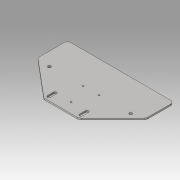
# Autodesk Inventor part: track side panel V1
Saved by Autodesk Inventor 2016 (Build 200138000, 138)
## iProperties
Created: 2015-10-10
Part Number: track side panel V1
Material: Generic
Document SubType Name: Modeling
Designer: Delta
Density: 1 g/cm^3
Appearance: Default
Author: Delta
Autodesk Inventor part; units mm, degrees
ref_plane "YZ Plane" through (0, 0, 0) normal (1, 0, 0) x (0, 1, 0)
ref_plane "XZ Plane" through (0, 0, 0) normal (0, 1, 0) x (-1, 0, 0)
ref_plane "XY Plane" through (0, 0, 0) normal (0, 0, 1) x (1, 0, 0)
sketch "Sketch1" plane through (0, 0, 0) normal (0, 1, 0) x (-1, 0, 0)
  line L0 (-77.6185, -139.5068) -> (-293.5185, -139.5068)
  line L1 (-293.5185, -139.5068) -> (-293.5185, -291.9068)
  line L2 (-293.5185, -291.9068) -> (-77.6185, -291.9068)
  line L3 (-77.6185, -291.9068) -> (-77.6185, -139.5068)
  point P0 (0, 0)
  dimension "d0" = 215.9
  dimension "d1" = 152.4
  constraints: 8 end point, 2 parallel, 1 horizontal, 1 perpendicular
  measures "d0" distance of L2.end L1.end
  measures "d1" distance of L1.end L0.end
extrude "Extrusion1" add sketch "Sketch1" along normal blind 3.175
sketch "Sketch2" plane through (0, 3.175, 0) normal (0, 1, 0) x (1, 0, 0)
  line L0 (77.6185, 291.9068) -> (77.6185, 139.5068) projected
  line L1 (77.6185, 139.5068) -> (293.5185, 139.5068) projected
  line L2 (293.5185, 139.5068) -> (293.5185, 291.9068) projected
  line L3 (293.5185, 291.9068) -> (77.6185, 291.9068) projected
  point P0 (0, 0)
  point P1 (156.9685, 165.5068)
  point P2 (104.9685, 218.5068)
  point P3 (269.9685, 218.5068)
  point P4 (221.9685, 165.5068)
  dimension "d4" = 144.35
  dimension "d5" = 26
  dimension "d7" = 79
  dimension "d19" = 27.35
  dimension "d20" = 79
  dimension "d21" = 26
  dimension "d22" = 79.35
  dimension "d23" = 192.35
  measures "d4" distance from line of L0 point (221.968, 165.507)
  measures "d5" distance from line of L1 point (221.968, 165.507)
  measures "d7" distance from line of L1 point (269.968, 218.507)
  measures "d19" distance from line of L0 point (104.968, 218.507)
  measures "d20" distance from line of L1 point (104.968, 218.507)
  measures "d21" distance from line of L1 point (156.968, 165.507)
  measures "d22" distance from line of L0 point (156.968, 165.507)
  measures "d23" distance from line of L0 point (269.968, 218.507)
hole "Hole1" at (156.9685, 3.175, -165.5068) at (104.9685, 3.175, -218.5068) at (269.9685, 3.175, -218.5068) at (221.9685, 3.175, -165.5068) direction (0, -1, 0) diameter 6 end through all
sketch "Sketch3" plane through (0, 3.175, 0) normal (0, 1, 0) x (1, 0, 0)
  line L0 (155.9994, 158.0068) -> (221.9685, 158.0068)
  circle A0 centre (221.9685, 165.5068) radius 3 projected
  circle A1 centre (104.3905, 218.5068) radius 3
  circle A2 centre (156.9685, 165.5068) radius 3 projected
  line L1 (153.2717, 158.9097) -> (79.8868, 220.4869)
  line L2 (77.6185, 139.5068) -> (293.5185, 139.5068)
  line L3 (293.5185, 229.1509) -> (293.5185, 276.0791)
  line L4 (293.5185, 291.9068) -> (77.6185, 291.9068)
  line L5 (77.6185, 291.9068) -> (77.6185, 139.5068)
  arc A3 (153.2717, 158.9097) -> (155.9994, 158.0068) centre (156.9685, 165.5068) ccw
  line L6 (96.6333, 206.4349) -> (77.6185, 222.3902)
  line L7 (48.2791, 233.5068) -> (391.5458, 233.5068) construction
  arc A4 (221.9685, 158.0068) -> (227.8466, 160.8487) centre (221.9685, 165.5068) ccw
  line L8 (227.8466, 160.8487) -> (291.6586, 224.6608)
  line L9 (293.5185, 226.5206) -> (293.5185, 282.4291)
  line L10 (293.5185, 139.5068) -> (293.5185, 291.9068) projected
  line L11 (287.1685, 282.4291) -> (83.9685, 282.4291)
  line L12 (77.6185, 276.0791) -> (77.6185, 225.3513)
  line L13 (77.6185, 291.9068) -> (77.6185, 139.5068) projected
  arc A5 (293.5185, 276.0791) -> (287.1685, 282.4291) centre (287.1685, 276.0791) ccw
  arc A6 (83.9685, 282.4291) -> (77.6185, 276.0791) centre (83.9685, 276.0791) ccw
  arc A7 (77.6185, 225.3513) -> (79.8868, 220.4869) centre (83.9685, 225.3513) ccw
  arc A8 (291.6586, 224.6608) -> (293.5185, 229.1509) centre (287.1685, 229.1509) ccw
  point P0 (0, 0)
  point P1 (77.6185, 282.4291)
  point P2 (77.6185, 160.8487)
  dimension "d24" = 7.5
  dimension "d40" = 98.7582
  dimension "d72" = 6
  dimension "d93" = 7.5
  dimension "d96" = 52.578
  dimension "d99" = 135
  dimension "d100" = 6.35
  dimension "d101" = 6.35
  dimension "d102" = 6.35
  dimension "d103" = 6.35
  dimension "d104" = 140
  constraints: 24 end point, 15 point on line, 12 point on circle, 8 tangent, 7 centre point, 4 horizontal, 2 coincident, 2 parallel, 1 collinear, 1 perpendicular
  measures "d24" distance from line of L0 A0.centre
  measures "d40" distance of L1.start L6.end
  measures "d72" diameter of A2
  measures "d93" radius of A4
  measures "d96" horizontal distance of A1.centre A3.centre
  measures "d99" angle of L0 L8
  measures "d100" radius of A5
  measures "d101" radius of A6
  measures "d102" radius of A7
  measures "d103" radius of A8
  measures "d104" angle of L0 L1
extrude "Extrusion3" cut sketch "Sketch3" against normal blind 25.4 contours L0 A4 L8 A8 L9 L10 L2 L5 L6 L1 A3 | L6 L5 A7 | A5 L11 A6 L5 L4 L10 L9
sketch "Sketch7" plane through (0, 3.175, 0) normal (0, 1, 0) x (1, 0, 0)
  circle A0 centre (156.9685, 165.5068) radius 3 projected
  line L0 (155.9994, 158.0068) -> (221.9685, 158.0068) projected
  circle A1 centre (156.9685, 178.0036) radius 2.9972
  line L1 (153.9713, 178.0036) -> (153.9713, 165.3773)
  line L2 (159.9657, 178.0043) -> (159.9685, 165.5075)
  circle A2 centre (221.9713, 178.0036) radius 2.9972
  circle A3 centre (221.9685, 165.5068) radius 3 projected
  line L3 (218.9741, 178.016) -> (218.9741, 165.3232)
  line L4 (224.9685, 178.0036) -> (224.9685, 165.5068)
  point P0 (0, 0)
  point P1 (218.9685, 165.5082)
  dimension "d76" = 5.9944
  dimension "d77" = 12.4968
  dimension "d78" = 5.9944
  dimension "d79" = 12.4968
  dimension "d88" = 6
  constraints: 9 point on circle, 8 end point, 3 vertical, 2 centre point, 1 tangent, 3 other
  measures "d76" diameter of A1
  measures "d77" distance of A0.centre A1.centre
  measures "d78" diameter of A2
  measures "d79" distance of A3.centre A2.centre
  measures "d88" diameter of A0
extrude "Extrusion4" cut sketch "Sketch7" against normal blind 25.4 contours A0 L1 A1 L2 | A1
sketch "Sketch8" plane through (0, 3.175, 0) normal (0, 1, 0) x (1, 0, 0)
  arc A0 (224.9685, 178.0036) -> (218.9741, 177.9913) centre (221.9713, 178.0036) ccw
  circle A1 centre (221.9685, 165.5068) radius 3
  line L0 (218.9741, 178.016) -> (218.9741, 165.3232)
  line L1 (224.9685, 178.0036) -> (224.9685, 165.5068)
  point P0 (0, 0)
  point P1 (218.9685, 165.5082)
  dimension "d82" = 5.9944
  dimension "d83" = 12.4968
  constraints: 6 point on circle, 4 end point, 2 centre point, 2 vertical, 1 point on line
  measures "d82" diameter of A0
  measures "d83" distance of A1.centre A0.centre
extrude "Extrusion5" cut sketch "Sketch8" against normal blind 25.4 contours L1 A1 L0 A0 | A1 L0 picked at (221.9464, 164.5591)
sketch "Sketch9" plane through (0, 3.175, 0) normal (0, 1, 0) x (1, 0, 0)
  point P0 (0, 0)
sketch "Sketch5" plane through (0, 3.175, 0) normal (0, 1, 0) x (1, 0, 0)
  circle A0 centre (104.9685, 218.5068) radius 3 projected
  circle A1 centre (104.9685, 218.5068) radius 22.225
  circle A2 centre (156.9685, 165.5068) radius 3 projected
  circle A3 centre (156.9685, 165.5068) radius 22.225
  circle A4 centre (221.9685, 165.5068) radius 3 projected
  circle A5 centre (221.9685, 165.5068) radius 22.225
  circle A6 centre (269.9685, 218.5068) radius 3 projected
  circle A7 centre (269.9685, 218.5068) radius 22.225
  line L0 (155.9994, 158.0068) -> (221.9685, 158.0068) projected
  line L1 (274.8943, 278.8204) -> (98.1742, 278.8204) projected
  arc A8 (224.9685, 178.0036) -> (218.9741, 178.016) centre (221.9713, 178.0036) ccw projected
  point P0 (0, 0)
  point P1 (205.7185, 218.5096)
  point P2 (189.4685, 178.0036)
  point P3 (173.2185, 218.5096)
  dimension "d45" = 44.45
  dimension "d47" = 44.45
  dimension "d48" = 44.45
  dimension "d49" = 44.45
  dimension "d50" = 60.5028
  dimension "d52" = 65
  dimension "d53" = 16.25
  dimension "d54" = 16.25
  dimension "d55" = 60.5028
  dimension "d58" = 52
  dimension "d62" = 32.5
  dimension "d95" = 60.3136
  dimension "d125" = 0
  constraints: 4 centre point, 4 coincident
  measures "d45" diameter of A1
  measures "d47" diameter of A3
  measures "d48" diameter of A5
  measures "d49" diameter of A7
  measures "d50" distance from line of L0 point (173.218, 218.51)
  measures "d52" distance of A5.centre A3.centre
  measures "d53" horizontal distance of point (173.218, 218.51) A3.centre
  measures "d54" horizontal distance of A5.centre point (205.718, 218.51)
  measures "d55" distance from line of L0 point (205.718, 218.51)
  measures "d58" horizontal distance of A3.centre A1.centre
  measures "d62" horizontal distance of A3.centre point (189.468, 178.004)
  measures "d95" distance from line of A1.centre L1
  measures "d125" vertical distance of A8.centre point (189.468, 178.004)
hole "Hole2" at (205.7185, 3.175, -218.5096) at (189.4685, 3.175, -178.0036) at (173.2185, 3.175, -218.5096) direction (0, -1, 0) diameter 3 end through all
sketch "Sketch11" plane through (0, 3.175, 0) normal (0, 1, 0) x (1, 0, 0)
  circle A0 centre (18.0131, 10.4316) radius 1.3525
  circle A1 centre (18.0131, 10.4316) radius 1.3525
  circle A2 centre (18.0131, 24.2612) radius 1.3525
  circle A3 centre (18.0131, 24.2612) radius 1.3525
  circle A4 centre (31.8426, 24.2612) radius 1.3525
  circle A5 centre (31.8426, 24.2612) radius 1.3525
  circle A6 centre (31.8426, 10.4316) radius 1.3525
  circle A7 centre (31.8426, 10.4316) radius 1.3525
  circle A8 centre (104.9685, 218.5068) radius 3 projected
  point P0 (0, 0)
  point P1 (24.9279, 17.3464)
  point P2 (24.9279, 17.3464)
  dimension "d126" = 13.8296
  dimension "d127" = 13.8296
  dimension "d128" = 6.9148
  dimension "d129" = 6.9148
  constraints: 8 centre point, 5 coincident
  measures "d126" distance of A3.centre A1.centre
  measures "d127" distance of A7.centre A1.centre
  measures "d128" horizontal distance of point (24.928, 17.346) A1.centre
  measures "d129" horizontal distance of point (24.928, 17.346) A3.centre
equation "\"d78\" = d76"
equation "\"d79\" = d77"
equation "\"d82\" = d84"
equation "\"d83\" = d85"
equation "\"d47\" = d45"
equation "\"d48\" = d45"
equation "\"d49\" = d48"
equation "\"d53\" = 0.25 * d52"
equation "\"d54\" = d53"
equation "\"d55\" = d50"
equation "\"d62\" = 0.5 * d52"
equation "\"d84\" = 5.9944"
equation "\"d85\" = 12.4968"
body "Solid1"
